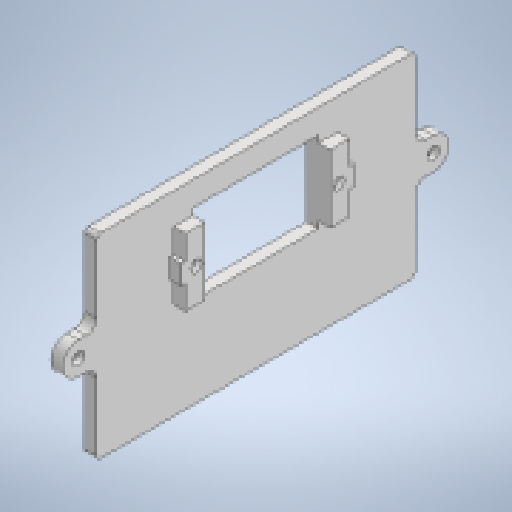
# Autodesk Inventor part: pokrywa_tyl
Saved by Autodesk Inventor 2023.4 (Build 274418000, 418)
## iProperties
Created: 2024-07-28
Part Number: pokrywa_tyl
Material: Ogólny
Document SubType Name: Modeling
Designer: kamil
Density: 1 g/cm^3
Appearance: Domyślna
Author: kamil
Autodesk Inventor part; units mm, degrees
ref_plane "YZ Plane" through (0, 0, 0) normal (1, 0, 0) x (0, 1, 0)
ref_plane "XZ Plane" through (0, 0, 0) normal (0, 1, 0) x (-1, 0, 0)
ref_plane "XY Plane" through (0, 0, 0) normal (0, 0, 1) x (1, 0, 0)
sketch "Szkic1" plane through (0, 0, 0) normal (1, 0, 0) x (0, 1, 0)
  line L0 (-29.4319, -23.6453) -> (19.8681, -23.6453)
  line L1 (19.8681, -23.6453) -> (19.8681, 56.9547)
  line L2 (19.8681, 56.9547) -> (-29.4319, 56.9547)
  line L3 (-29.4319, 56.9547) -> (-29.4319, -23.6453)
  point P0 (0, 0)
  dimension "d0" = 80.6
  dimension "d1" = 49.3
  constraints: 8 end point, 2 parallel, 1 horizontal, 1 perpendicular
  measures "d0" distance of L0.end L1.end
  measures "d1" distance between parallel lines of L3 L1
extrude "Wyciągnięcie proste1" add sketch "Szkic1" along normal blind 3
sketch "Sketch6" plane through (0, 0, 0) normal (-1, 0, 0) x (0, 0, 1)
  arc A0 (-28.0945, -0.5319) -> (-28.0945, -9.0319) centre (-28.0945, -4.7819) ccw
  line L0 (-26.3445, -9.0319) -> (-28.0945, -9.0319)
  line L1 (-26.3445, -0.5319) -> (-28.0945, -0.5319)
  line L2 (59.654, -9.0319) -> (61.404, -9.0319)
  arc A1 (61.404, -9.0319) -> (61.404, -0.5319) centre (61.404, -4.7819) ccw
  line L3 (59.654, -0.5319) -> (61.404, -0.5319)
  line L4 (-23.6453, 19.8681) -> (56.9547, 19.8681)
  line L5 (-23.6453, -29.4319) -> (-23.6453, 19.8681)
  line L6 (56.9547, -29.4319) -> (-23.6453, -29.4319)
  line L7 (56.9547, 19.8681) -> (56.9547, -29.4319)
  line L8 (-26.3445, -8.7819) -> (-28.0945, -8.7819)
  arc A2 (-28.0945, -0.7819) -> (-28.0945, -8.7819) centre (-28.0945, -4.7819) ccw
  line L9 (-28.0945, -0.7819) -> (-26.3445, -0.7819)
  line L10 (59.654, -0.7819) -> (61.404, -0.7819)
  arc A3 (61.404, -8.7819) -> (61.404, -0.7819) centre (61.404, -4.7819) ccw
  line L11 (61.404, -8.7819) -> (59.654, -8.7819)
  line L12 (-26.3445, -0.7819) -> (-23.6453, -0.7819)
  line L13 (-23.6453, -29.4319) -> (-23.6453, 19.8681)
  line L14 (-26.3445, -8.7819) -> (-23.6453, -8.7819)
  line L15 (59.654, -0.7819) -> (56.9547, -0.7819)
  line L16 (59.654, -8.7819) -> (56.9547, -8.7819)
  point P0 (0, 0)
extrude "Extrusion4" add sketch "Sketch6" against normal blind 3 contours L5 L14 L8 A2 L9 L12 | L15 L10 A3 L11 L16 L7
fillet "Fillet2" radius 2.5 4 edges at (1.5, -0.7819, -23.6453) (1.5, -8.7819, -23.6453) (1.5, -0.7819, 56.9547) (1.5, -8.7819, 56.9547)
sketch "Sketch7" plane through (0, 0, 0) normal (-1, 0, 0) x (0, 0, 1)
  arc A0 (-28.0945, -0.7819) -> (-28.0945, -8.7819) centre (-28.0945, -4.7819) ccw projected
  arc A1 (61.404, -8.7819) -> (61.404, -0.7819) centre (61.404, -4.7819) ccw projected
  point P0 (0, 0)
hole "Hole3" at (0, -4.7819, -28.0945) at (0, -4.7819, 61.404) direction (1, 0, 0) diameter 3.2 depth 3 countersink diameter 6 countersink angle 90
fillet "Fillet3" radius 1 4 edges at (1.5, 19.8681, -23.6453) (1.5, 19.8681, 56.9547) (1.5, -29.4319, -23.6453) (1.5, -29.4319, 56.9547)
sketch "Sketch8" plane through (0, 0, 0) normal (-1, 0, 0) x (0, 0, 1)
  line L0 (32.3929, 13.5523) -> (1.0929, 13.5523) projected
  line L1 (1.0929, 13.5523) -> (1.0929, -6.4477) projected
  line L2 (1.0929, -6.4477) -> (32.3929, -6.4477) projected
  line L3 (32.3929, -6.4477) -> (32.3929, 13.5523) projected
  line L4 (0.8929, -6.6477) -> (0.8929, 13.7523)
  line L5 (0.8929, 13.7523) -> (32.5929, 13.7523)
  line L6 (32.5929, 13.7523) -> (32.5929, -6.6477)
  line L7 (32.5929, -6.6477) -> (0.8929, -6.6477)
  point P0 (0, 0)
  dimension "d38" = 0.2
  constraints: 8 end point, 3 other
  measures "d38" distance between parallel lines of L1 L4
extrude "Extrusion5" cut sketch "Sketch8" against normal blind 3 contours L3 L2 L1 L0 | L4 L5 L6 L7
sketch "Sketch9" plane through (3, 0, 0) normal (1, 0, 0) x (0, 0, -1)
  line L0 (-32.5929, 13.7523) -> (-0.8929, 13.7523) projected
  line L1 (-0.8929, 13.7523) -> (-0.8929, -6.6477) projected
  line L2 (-0.8929, -6.6477) -> (-32.5929, -6.6477) projected
  line L3 (-32.5929, -6.6477) -> (-32.5929, 13.7523) projected
  circle A0 centre (28.0945, -4.7819) radius 1.6 projected
  circle A1 centre (-61.404, -4.7819) radius 1.6 projected
  arc A2 (-56.9547, -28.4319) -> (-55.9547, -29.4319) centre (-55.9547, -28.4319) ccw projected
  line L4 (-55.9547, -29.4319) -> (22.6453, -29.4319) projected
  arc A3 (22.6453, -29.4319) -> (23.6453, -28.4319) centre (22.6453, -28.4319) ccw projected
  line L5 (23.6453, -28.4319) -> (23.6453, -11.2819) projected
  arc A4 (26.1453, -8.7819) -> (23.6453, -11.2819) centre (26.1453, -11.2819) ccw projected
  line L6 (26.1453, -8.7819) -> (28.0945, -8.7819) projected
  arc A5 (28.0945, -8.7819) -> (28.0945, -0.7819) centre (28.0945, -4.7819) ccw projected
  line L7 (28.0945, -0.7819) -> (26.1453, -0.7819) projected
  arc A6 (23.6453, 1.7181) -> (26.1453, -0.7819) centre (26.1453, 1.7181) ccw projected
  line L8 (23.6453, 1.7181) -> (23.6453, 18.8681) projected
  arc A7 (23.6453, 18.8681) -> (22.6453, 19.8681) centre (22.6453, 18.8681) ccw projected
  line L9 (22.6453, 19.8681) -> (-55.9547, 19.8681) projected
  arc A8 (-55.9547, 19.8681) -> (-56.9547, 18.8681) centre (-55.9547, 18.8681) ccw projected
  line L10 (-56.9547, 18.8681) -> (-56.9547, 1.7181) projected
  arc A9 (-59.4547, -0.7819) -> (-56.9547, 1.7181) centre (-59.4547, 1.7181) ccw projected
  line L11 (-59.4547, -0.7819) -> (-61.404, -0.7819) projected
  arc A10 (-61.404, -0.7819) -> (-61.404, -8.7819) centre (-61.404, -4.7819) ccw projected
  line L12 (-61.404, -8.7819) -> (-59.4547, -8.7819) projected
  arc A11 (-56.9547, -11.2819) -> (-59.4547, -8.7819) centre (-59.4547, -11.2819) ccw projected
  line L13 (-56.9547, -11.2819) -> (-56.9547, -28.4319) projected
  line L14 (-37.4929, 12.0523) -> (-37.4929, 6.0523) projected
  line L15 (-37.4929, 6.0523) -> (-38.4929, 6.0523) projected
  line L16 (-38.4929, 6.0523) -> (-38.4929, 1.0523) projected
  line L17 (-38.4929, 1.0523) -> (-37.4929, 1.0523) projected
  line L18 (-37.4929, 1.0523) -> (-37.4929, -4.9477) projected
  line L19 (-37.4929, -4.9477) -> (4.0071, -4.9477) projected
  line L20 (4.0071, -4.9477) -> (4.0071, 1.0523) projected
  line L21 (4.0071, 1.0523) -> (5.0071, 1.0523) projected
  line L22 (5.0071, 1.0523) -> (5.0071, 6.0523) projected
  line L23 (5.0071, 6.0523) -> (4.0071, 6.0523) projected
  line L24 (4.0071, 6.0523) -> (4.0071, 12.0523) projected
  line L25 (4.0071, 12.0523) -> (-37.4929, 12.0523) projected
  circle A12 centre (1.2571, 3.5523) radius 1.2 projected
  circle A13 centre (-34.7429, 3.5523) radius 1.2 projected
  point P0 (0, 0)
  point P1 (-0.8929, 12.0523)
  point P2 (-0.8929, -4.9477)
  point P3 (-32.5929, -4.9477)
  point P4 (-32.5929, 12.0523)
ref_plane "Work Plane2" through (6, -4.9477, 32.3929) normal (-1, 0, 0) x (0, 0, 1)
extrude "Extrusion6" add sketch "Sketch9" along normal up to surface (3 mm away) contours L3 L19 L18 L17 L16 L15 L14 L25 | L25 L24 L23 L22 L21 L20 L19 L1 | A12 | A13
sketch "Sketch10" plane through (6, -4.9477, 32.5929) normal (1, 0, 0) x (0, 0, -1)
  circle A0 centre (33.85, 8.5) radius 1.2 projected
  circle A1 centre (-2.15, 8.5) radius 1.2 projected
  point P0 (32.5929, 4.9477)
hole "Hole4" at (6, 3.5523, -1.2571) at (6, 3.5523, 34.7429) direction (-1, 0, 0) diameter 1.5 depth 5 tip angle 118 countersink diameter 3 countersink angle 90
sketch "Sketch11" plane through (3, 0, 0) normal (1, 0, 0) x (0, 0, -1)
  arc A0 (-56.9547, -28.4319) -> (-55.9547, -29.4319) centre (-55.9547, -28.4319) ccw projected
  line L0 (-55.9547, -29.4319) -> (22.6453, -29.4319) projected
  arc A1 (22.6453, -29.4319) -> (23.6453, -28.4319) centre (22.6453, -28.4319) ccw projected
  line L1 (23.6453, -28.4319) -> (23.6453, -11.2819) projected
  arc A2 (26.1453, -8.7819) -> (23.6453, -11.2819) centre (26.1453, -11.2819) ccw projected
  line L2 (26.1453, -8.7819) -> (28.0945, -8.7819) projected
  arc A3 (28.0945, -8.7819) -> (28.0945, -0.7819) centre (28.0945, -4.7819) ccw projected
  line L3 (28.0945, -0.7819) -> (26.1453, -0.7819) projected
  arc A4 (23.6453, 1.7181) -> (26.1453, -0.7819) centre (26.1453, 1.7181) ccw projected
  line L4 (23.6453, 1.7181) -> (23.6453, 18.8681) projected
  arc A5 (23.6453, 18.8681) -> (22.6453, 19.8681) centre (22.6453, 18.8681) ccw projected
  line L5 (22.6453, 19.8681) -> (-55.9547, 19.8681) projected
  arc A6 (-55.9547, 19.8681) -> (-56.9547, 18.8681) centre (-55.9547, 18.8681) ccw projected
  line L6 (-56.9547, 18.8681) -> (-56.9547, 1.7181) projected
  arc A7 (-59.4547, -0.7819) -> (-56.9547, 1.7181) centre (-59.4547, 1.7181) ccw projected
  line L7 (-59.4547, -0.7819) -> (-61.404, -0.7819) projected
  arc A8 (-61.404, -0.7819) -> (-61.404, -8.7819) centre (-61.404, -4.7819) ccw projected
  line L8 (-61.404, -8.7819) -> (-59.4547, -8.7819) projected
  arc A9 (-56.9547, -11.2819) -> (-59.4547, -8.7819) centre (-59.4547, -11.2819) ccw projected
  line L9 (-56.9547, -11.2819) -> (-56.9547, -28.4319) projected
  circle A10 centre (-61.404, -4.7819) radius 1.6 projected
  circle A11 centre (28.0945, -4.7819) radius 1.6 projected
  line L10 (-0.8929, 12.0523) -> (4.0071, 12.0523) projected
  line L11 (4.0071, 12.0523) -> (4.0071, 6.0523) projected
  line L12 (4.0071, 6.0523) -> (5.0071, 6.0523) projected
  line L13 (5.0071, 6.0523) -> (5.0071, 1.0523) projected
  line L14 (5.0071, 1.0523) -> (4.0071, 1.0523) projected
  line L15 (4.0071, 1.0523) -> (4.0071, -4.9477) projected
  line L16 (4.0071, -4.9477) -> (-0.8929, -4.9477) projected
  line L17 (-0.8929, -4.9477) -> (-0.8929, -6.6477) projected
  line L18 (-0.8929, -6.6477) -> (-32.5929, -6.6477) projected
  line L19 (-32.5929, -6.6477) -> (-32.5929, -4.9477) projected
  line L20 (-32.5929, -4.9477) -> (-37.4929, -4.9477) projected
  line L21 (-37.4929, -4.9477) -> (-37.4929, 1.0523) projected
  line L22 (-37.4929, 1.0523) -> (-38.4929, 1.0523) projected
  line L23 (-38.4929, 1.0523) -> (-38.4929, 6.0523) projected
  line L24 (-38.4929, 6.0523) -> (-37.4929, 6.0523) projected
  line L25 (-37.4929, 6.0523) -> (-37.4929, 12.0523) projected
  line L26 (-37.4929, 12.0523) -> (-32.5929, 12.0523) projected
  line L27 (-32.5929, 12.0523) -> (-32.5929, 13.7523) projected
  line L28 (-32.5929, 13.7523) -> (-0.8929, 13.7523) projected
  line L29 (-0.8929, 13.7523) -> (-0.8929, 12.0523) projected
  line L30 (-41.6988, -13.0398) -> (-26.6988, -13.0398)
  line L31 (-26.6988, -13.0398) -> (-26.6988, -23.0398)
  line L32 (-26.6988, -23.0398) -> (-41.6988, -23.0398)
  line L33 (-41.6988, -23.0398) -> (-41.6988, -13.0398)
  line L34 (-10.6988, -18.0398) -> (-0.6988, -18.0398) construction
  line L35 (-10.6988, -22.0398) -> (-0.6988, -22.0398)
  line L36 (-0.6988, -14.0398) -> (-10.6988, -14.0398)
  arc A12 (-10.6988, -14.0398) -> (-10.6988, -22.0398) centre (-10.6988, -18.0398) ccw
  arc A13 (-0.6988, -22.0398) -> (-0.6988, -14.0398) centre (-0.6988, -18.0398) ccw
  line L37 (-26.6988, -18.0398) -> (-6.6988, -18.0398) construction
  line L38 (-0.8929, -6.6477) -> (-32.5929, -6.6477) construction
  line L39 (-16.7429, -6.6477) -> (-16.6547, -29.4319) construction
  line L40 (-55.9547, -29.4319) -> (22.6453, -29.4319) construction
  point P0 (0, 0)
  point P1 (-5.6988, -18.0398)
  point P2 (-16.6988, -18.0398)
  dimension "d50" = 10
  dimension "d51" = 15
  dimension "d53" = 20
  dimension "d54" = 10
  dimension "d55" = 8
  constraints: 20 end point, 6 midpoint, 5 point on circle, 4 parallel, 4 tangent, 2 centre point, 2 horizontal, 1 perpendicular
  measures "d50" distance between parallel lines of L32 L30
  measures "d51" distance between parallel lines of L31 L33
  measures "d53" distance of L37.start L37.end
  measures "d54" distance of L34.start L34.end
  measures "d55" distance between parallel lines of L35 L36
extrude "Extrusion7" cut sketch "Sketch11" against normal through all contours L30 L31 L32 L33 | A12 L36 A13 L35
